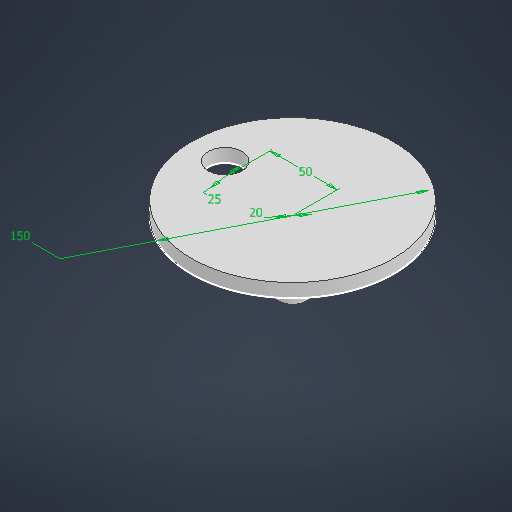
# Autodesk Inventor part: top
Saved by Autodesk Inventor 2025.1 (Build 291241000, 241)
## iProperties
Created: 2025-02-19
Part Number: top
Material: Generic
Document SubType Name: Modeling
Designer: jerem
Density: 1 g/cm^3
Appearance: Default
Author: jerem
Autodesk Inventor part; units mm, degrees
ref_plane "YZ Plane" through (0, 0, 0) normal (1, 0, 0) x (0, 1, 0)
ref_plane "XZ Plane" through (0, 0, 0) normal (0, 1, 0) x (-1, 0, 0)
ref_plane "XY Plane" through (0, 0, 0) normal (0, 0, 1) x (1, 0, 0)
sketch "Sketch1" plane through (0, 0, 0) normal (0, 1, 0) x (-1, 0, 0)
  circle A0 centre (0, 0) radius 75
  circle A1 centre (50, 0) radius 12.5
  line L0 (0, 0) -> (50, 0) construction
  circle A2 centre (0, 0) radius 10
  dimension "d4" = 150
  dimension "d5" = 25
  dimension "d6" = 50
  dimension "d7" = 20
  constraints: 3 centre point, 3 coincident, 2 end point, 1 horizontal
  measures "d4" diameter of A0
  measures "d5" diameter of A1
  measures "d6" distance of point (0, 0) A1.centre
  measures "d7" diameter of A2
extrude "Extrusion1" add sketch "Sketch1" along normal blind 10 contours A0 | A2
extrude "Extrusion2" add sketch "Sketch1" against normal blind 50 contours A2
body "Solid1"
